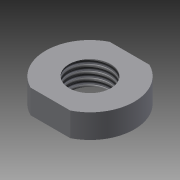
# Autodesk Inventor part: BallBearingConeLockNut
Saved by Autodesk Inventor 2015 (Build 190159000, 159)
## iProperties
Created: 2017-01-14
Part Number: BallBearingConeLockNut
Material: Generic
Document SubType Name: Modeling
Designer: 1esh9
Density: 1 g/cm^3
Appearance: Default
Author: 1esh9
Autodesk Inventor part; units mm, degrees
ref_plane "YZ Plane" through (0, 0, 0) normal (1, 0, 0) x (0, 1, 0)
ref_plane "XZ Plane" through (0, 0, 0) normal (0, 1, 0) x (-1, 0, 0)
ref_plane "XY Plane" through (0, 0, 0) normal (0, 0, 1) x (1, 0, 0)
sketch "Sketch1" plane through (0, 0, 0) normal (0, 0, 1) x (1, 0, 0)
  circle A0 centre (0, 0) radius 4.435
  line L0 (-4.2273, 8.435) -> (4.2273, 8.435)
  line L1 (-4.2273, -8.435) -> (4.2273, -8.435)
  arc A1 (-4.2273, 8.435) -> (-4.2273, -8.435) centre (0, 0) ccw
  arc A2 (4.2273, -8.435) -> (4.2273, 8.435) centre (0, 0) ccw
  dimension "d0" = 8.87
  dimension "d2" = 16.87
  dimension "d3" = 8.435
  constraints: 4 end point, 4 point on circle, 3 centre point, 2 coincident, 2 horizontal
  measures "d0" diameter of A0
  measures "d2" distance between parallel lines of L1 L0
  measures "d3" distance from line of point (0, 0) L0
extrude "Extrusion1" add sketch "Sketch1" along normal blind 5.1
thread "Thread1" size "M9x1.25" class "6H" standard "ANSI Metric M Profile" full length
equation "\"d3\" = 0.5 * d2"
body "Solid1"
